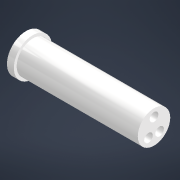
# Autodesk Inventor part: 029
Saved by Autodesk Inventor 2022 (Build 260153000, 153)
## iProperties
Created: 2022-04-04
Part Number: 029
Material: Acetal Resin, White
Document SubType Name: Modeling
Designer: Vinicius Miguel
Density: 1.425 g/cm^3
Appearance: Smooth - White
Mass: 23.4979 g
Surface Area: 85.2942 cm^2
Volume: 16.4897 cm^3
Author: Vinicius Miguel
Autodesk Inventor part; units mm, degrees
ref_plane "YZ Plane" through (0, 0, 0) normal (1, 0, 0) x (0, 1, 0)
ref_plane "XZ Plane" through (0, 0, 0) normal (0, 1, 0) x (-1, 0, 0)
ref_plane "XY Plane" through (0, 0, 0) normal (0, 0, 1) x (1, 0, 0)
sketch "Sketch1" plane through (0, 0, 0) normal (0, 1, 0) x (-1, 0, 0)
  line L0 (0, 0) -> (74, 0)
  line L1 (74, 0) -> (74, -11)
  line L2 (74, -11) -> (70, -11)
  line L3 (70, -11) -> (70, -9.375)
  line L4 (70, -9.375) -> (0, -9.375)
  line L5 (0, -9.375) -> (0, 0)
  dimension "d0" = 18.75
  dimension "d1" = 70
  dimension "d2" = 22
  dimension "d3" = 4
  constraints: 12 end point, 5 perpendicular, 1 horizontal
  measures "d0" diameter of L4 L0
  measures "d1" distance of L3.end L4.end
  measures "d2" diameter of L2 L0
  measures "d3" distance of L1.end L2.end
revolve "Revolution1" add sketch "Sketch1" angle 360 about axis through (0, 0, 0) along (-1, 0, 0)
sketch "Sketch2" plane through (0, 0, 0) normal (1, 0, 0) x (0, 0, -1)
  circle A0 centre (0, 0) radius 5
  line L0 (0, 0) -> (-5, 0)
  line L1 (0, 0) -> (-3.2139, -3.8302)
  point P0 (0, 5)
  point P1 (3.2139, -3.8302)
  dimension "d5" = 10
  dimension "d6" = 50
  constraints: 4 end point, 4 point on circle, 1 centre point, 1 coincident, 1 horizontal, 1 horizontal alignment, 1 vertical alignment
  measures "d5" diameter of A0
  measures "d6" angle of L0 L1
hole "Hole1" at (0, 5, 0) at (0, -3.8302, 3.2139) at (0, -3.8302, -3.2139) direction (-1, 0, 0) diameter 5 end through all
body "Solid1"
